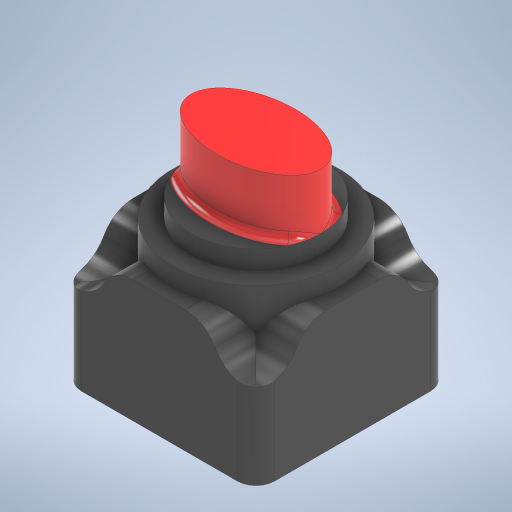
# Autodesk Inventor part: Voltage Cutoff Switch
Saved by Autodesk Inventor 2023 (Build 270158000, 158)
## iProperties
Created: 2022-07-16
Part Number: Voltage Cutoff Switch
Material: Generic
Document SubType Name: Modeling
Designer: justi
Density: 1 g/cm^3
Appearance: 192,192,192
Author: justi
Autodesk Inventor part; units mm, degrees
ref_plane "YZ Plane" through (0, 0, 0) normal (1, 0, 0) x (0, 1, 0)
ref_plane "XZ Plane" through (0, 0, 0) normal (0, 1, 0) x (-1, 0, 0)
ref_plane "XY Plane" through (0, 0, 0) normal (0, 0, 1) x (1, 0, 0)
sketch "Sketch1" plane through (0, 0, 0) normal (0, 1, 0) x (-1, 0, 0)
  line L0 (0, 0) -> (66.04, 0)
  line L1 (66.04, 0) -> (66.04, -66.04)
  line L2 (66.04, -66.04) -> (0, -66.04)
  line L3 (0, -66.04) -> (0, 0)
  dimension "d0" = 66.04
  dimension "d1" = 66.04
  constraints: 8 end point, 2 parallel, 1 horizontal, 1 perpendicular
  measures "d0" distance of L0.end L1.end
  measures "d1" distance of L1.end L2.end
extrude "Extrusion1" add sketch "Sketch1" along normal blind 73.66
sketch "Sketch2" plane through (0, 73.66, 0) normal (0, 1, 0) x (1, 0, 0)
  circle A0 centre (-33.02, 33.02) radius 31.75
  line L0 (0, 0) -> (0, 66.04) projected
  line L1 (0, 66.04) -> (-66.04, 66.04) projected
  line L2 (-66.04, 0) -> (0, 0) projected
  line L3 (-66.04, 66.04) -> (0, 66.04)
  line L4 (0, 66.04) -> (0, 0)
  line L5 (0, 0) -> (-66.04, 0)
  line L6 (-66.04, 0) -> (-66.04, 66.04)
  dimension "d4" = 63.5
  dimension "d5" = 33.02
  dimension "d6" = 33.02
  constraints: 8 end point, 2 parallel, 1 centre point, 1 horizontal, 1 perpendicular
  measures "d4" diameter of A0
  measures "d5" distance from line of L0 A0.centre
  measures "d6" distance from line of L1 A0.centre
extrude "Extrusion2" cut sketch "Sketch2" against normal blind 25.4
sketch "Sketch3" plane through (-33.02, 73.66, -33.02) normal (0, 1, 0) x (1, 0, 0)
  circle A0 centre (0, 0) radius 28.575
  circle A1 centre (0, 0) radius 31.75
  point P0 (33.02, -33.02)
  dimension "d9" = 57.15
  constraints: 2 centre point, 1 coincident
  measures "d9" diameter of A0
extrude "Extrusion3" cut sketch "Sketch3" against normal blind 25.4
sketch "Sketch4" plane through (-33.02, 73.66, -33.02) normal (0, 1, 0) x (1, 0, 0)
  circle A0 centre (0, 0) radius 25.0031
  circle A1 centre (0, 0) radius 22.225
  circle A2 centre (0, 0) radius 28.575
  point P0 (33.02, -33.02)
  dimension "d12" = 44.45
  constraints: 3 centre point, 2 coincident
  measures "d12" diameter of A1
extrude "Extrusion4" cut sketch "Sketch4" against normal blind 19.05 contours A0 | A2
sketch "Sketch5" plane through (0, 48.26, 0) normal (0, 1, 0) x (1, 0, 0)
  line L0 (-66.04, 0) -> (0, 0) projected
  line L1 (0, 0) -> (-12.7, 0)
  line L2 (-12.7, 0) -> (-12.7, 12.7)
  line L3 (-12.7, 12.7) -> (0, 12.7)
  line L4 (0, 12.7) -> (0, 0)
  line L5 (-66.04, 66.04) -> (-66.04, 0) projected
  line L6 (-66.04, 0) -> (-53.34, 0)
  line L7 (-53.34, 0) -> (-53.34, 12.7)
  line L8 (-53.34, 12.7) -> (-66.04, 12.7)
  line L9 (-66.04, 12.7) -> (-66.04, 0)
  line L10 (0, 66.04) -> (-66.04, 66.04) projected
  line L11 (-66.04, 66.04) -> (-53.34, 66.04)
  line L12 (-53.34, 66.04) -> (-53.34, 53.34)
  line L13 (-53.34, 53.34) -> (-66.04, 53.34)
  line L14 (-66.04, 53.34) -> (-66.04, 66.04)
  line L15 (0, 0) -> (0, 66.04) projected
  line L16 (0, 66.04) -> (-12.7, 66.04)
  line L17 (-12.7, 66.04) -> (-12.7, 53.34)
  line L18 (-12.7, 53.34) -> (0, 53.34)
  line L19 (0, 53.34) -> (0, 66.04)
  point P0 (0, 53.34)
  dimension "d15" = 12.7
  dimension "d16" = 12.7
  dimension "d17" = 12.7
  dimension "d18" = 12.7
  dimension "d19" = 12.7
  dimension "d20" = 12.7
  dimension "d21" = 12.7
  dimension "d22" = 12.7
  constraints: 32 end point, 8 parallel, 4 horizontal, 4 perpendicular
  measures "d15" distance of L1.end L2.end
  measures "d16" distance of L2.end L3.end
  measures "d17" distance of L8.end L7.end
  measures "d18" distance of L6.end L7.end
  measures "d19" distance of L12.end L13.end
  measures "d20" distance of L11.end L12.end
  measures "d21" distance of L16.end L17.end
  measures "d22" distance of L17.end L18.end
extrude "Extrusion5" cut sketch "Sketch5" against normal blind 12.7 contours L5 L8 L7 L0 | L2 L3 L4 L0 | L5 L10 L12 L13 | L18 L17 L10 L15
fillet "Fillet1" radius 6.35 4 edges at (-66.04, 17.78, -66.04) (0, 17.78, -66.04) (-66.04, 17.78, 0) (0, 17.78, 0)
fillet "Fillet2" radius 11.43 8 edges at (-53.34, 48.26, -59.69) (-59.69, 48.26, -53.34) (-59.69, 48.26, -12.7) (-53.34, 48.26, -6.35) (-12.7, 48.26, -6.35) (-6.35, 48.26, -12.7) (-6.35, 48.26, -53.34) (-12.7, 48.26, -59.69)
fillet "Fillet3" radius 12.7 8 edges at (-6.35, 35.56, -53.34) (-12.7, 35.56, -59.69) (-59.69, 35.56, -53.34) (-53.34, 35.56, -59.69) (-12.7, 35.56, -6.35) (-6.35, 35.56, -12.7) (-59.69, 35.56, -12.7) (-53.34, 35.56, -6.35)
sketch "Sketch6" plane through (0, 0, -6.35) normal (1, 0, 0) x (0, 0, -1)
  line L0 (0, 0) -> (-6.35, 0) projected
  line L1 (-6.35, 0) -> (81.8733, 0)
  line L2 (81.8733, 0) -> (81.8733, 6.35)
  line L3 (81.8733, 6.35) -> (-6.35, 6.35)
  line L4 (-6.35, 6.35) -> (-6.35, 0)
  dimension "d28" = 6.35
  constraints: 8 end point, 2 parallel, 1 horizontal, 1 perpendicular
  measures "d28" distance of L1.end L2.end
extrude "Extrusion6" cut sketch "Sketch6" against normal blind 127
sketch "Sketch7" plane through (-33.02, 73.66, -33.02) normal (0, 1, 0) x (1, 0, 0)
  circle A0 centre (0, 0) radius 22.225
  point P0 (33.02, -33.02)
  constraints: 1 centre point
extrude "Extrusion7" add sketch "Sketch7" along normal blind 6.35
sketch "Sketch8" plane through (-33.02, 80.01, -33.02) normal (0, 1, 0) x (1, 0, 0)
  ellipse E0 centre (0, 0) end of major axis (-22.225, 0) minor radius 13.3612
  circle A0 centre (0, 0) radius 22.225
  point P0 (33.02, -33.02)
  point P1 (22.225, 0)
  point P2 (-22.225, 0)
  constraints: 1 centre point, 1 coincident, 2 other
extrude "Extrusion8" cut sketch "Sketch8" against normal blind 19.05 contours A0 E0 | E0 A0
fillet "Fillet4" radius 2.54 2 edges at (-33.02, 60.96, -46.3812) (-33.02, 60.96, -19.6588)
body "Solid1"
